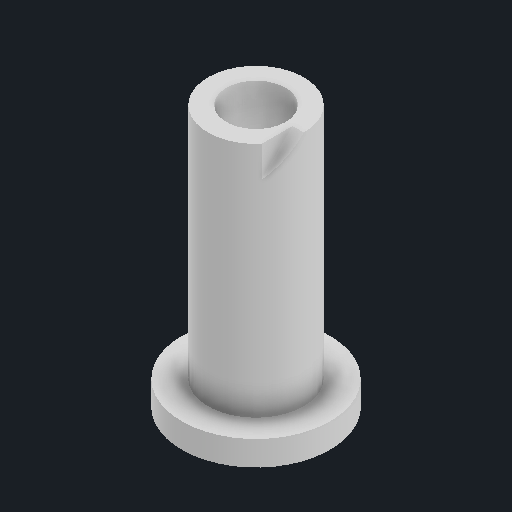
# Autodesk Inventor part: Штырь
Saved by Autodesk Inventor 2026.2 (Build 302298000, 298)
## iProperties
Created: 2026-02-19
Part Number: Штырь
Material: Типовые
Document SubType Name: Modeling
Designer: Leonid
Density: 1 g/cm^3
Appearance: По умолчанию
Author: Leonid
Autodesk Inventor part; units mm, degrees
ref_plane "XZ Plane" through (0, 0, 0) normal (0, 1, 0) x (-1, 0, 0)
ref_plane "XY Plane" through (0, 0, 0) normal (0, 0, 1) x (1, 0, 0)
sketch "Эскиз1" plane through (0, 0, 0) normal (0, 1, 0) x (-1, 0, 0)
  circle A0 centre (0, 0) radius 3.75
  circle A1 centre (0, 0) radius 2.425
  circle A2 centre (0, 0) radius 1.5
  dimension "d0" = 4.85
  dimension "d1" = 7.5
  dimension "d2" = 3
  constraints: 3 centre point, 3 coincident
  measures "d0" diameter of A1
  measures "d1" diameter of A0
  measures "d2" diameter of A2
extrude "Выдавливание1" add sketch "Эскиз1" along normal blind 12 contours A1
extrude "Выдавливание2" add sketch "Эскиз1" against normal blind 1.25 contours A0 | A1
ref_plane "РабПлоскость1" through (1.85, 0, 0) normal (1, 0, 0) x (0, 1, 0)
sketch "Эскиз2" plane through (1.85, 0, 0) normal (1, 0, 0) x (0, 1, 0)
  line L0 (12, -2.425) -> (12, 2.425) projected
  line L1 (0, -2.425) -> (0, 2.425) projected
  line L2 (12, -2.425) -> (12, 2.425) projected
  line L3 (0, -2.425) -> (0, 2.425) projected
  line L4 (12, 0) -> (9.575, 2.425)
  line L5 (0, 2.425) -> (12, 2.425) projected
  line L6 (12, 0) -> (15.4295, 0) construction
  line L7 (9.575, 2.425) -> (12, 2.425)
  point P0 (0, 0)
  dimension "d8" = 135
  constraints: 6 end point, 1 collinear, 1 equal length, 1 horizontal, 1 midpoint, 1 point on line
  measures "d8" angle of L6 L4
extrude "Выдавливание3" cut sketch "Эскиз2" along normal blind 10
